GridUp-PCB (Autodesk Fusion 360 design; units mm, degrees)
part number: 2026-09-14-08-15-55-205
Autodesk Fusion 360 part; units mm, degrees
sketch "Çizim257" plane through (0, 0, 0) normal (0, 0, 1) x (1, 0, 0)
  line L0 (0, 0) -> (110, 0)
  line L1 (110, 0) -> (110, 70)
  line L2 (110, 70) -> (0, 70)
  line L3 (0, 70) -> (0, 0)
extrude "Ekstrüzyon257" add sketch "Çizim257" along normal blind 1.6 makes body 1
fillet "Kavis8" radius 2 4 edges at (0, 70, 0.8) (110, 70, 0.8) (110, 0, 0.8) (0, 0, 0.8) on bodies 1
sketch "Çizim258" plane through (0, 0, 0) normal (0, 0, 1) x (1, 0, 0)
  circle A0 centre (7, 7) radius 1.6
  circle A1 centre (103, 7) radius 1.6
  circle A2 centre (7, 63) radius 1.6
  circle A3 centre (103, 63) radius 1.6
  line L0 (81.5, -1) -> (82.5, -1)
  line L1 (82.5, -1) -> (82.5, 40)
  line L2 (82.5, 40) -> (81.5, 40)
  line L3 (81.5, 40) -> (81.5, -1)
  circle A4 centre (0, 0) radius 4
  circle A5 centre (110, 0) radius 4
  circle A6 centre (0, 70) radius 4
  circle A7 centre (110, 70) radius 4
extrude "Ekstrüzyon258" cut sketch "Çizim258" along normal mid plane 10 bodies 1
ref_plane "WorkPlane238" through (0, 0, 1.6) normal (0, 0, 1) x (1, 0, 0)
sketch "Çizim259" plane through (0, 0, 1.6) normal (0, 0, 1) x (1, 0, 0)
  circle A0 centre (55, 37.5) radius 4.65
extrude "Ekstrüzyon259" add sketch "Çizim259" along normal blind 6 separate body makes body 2
ref_plane "WorkPlane239" through (0, 0, 1.6) normal (0, 0, 1) x (1, 0, 0)
sketch "Çizim260" plane through (0, 0, 1.6) normal (0, 0, 1) x (1, 0, 0)
  line L0 (5.75, 29.75) -> (8.25, 29.75)
  line L1 (8.25, 29.75) -> (8.25, 32.25)
  line L2 (8.25, 32.25) -> (5.75, 32.25)
  line L3 (5.75, 32.25) -> (5.75, 29.75)
extrude "Ekstrüzyon260" add sketch "Çizim260" along normal blind 0.9 separate body makes body 3
ref_plane "WorkPlane240" through (0, 0, 1.6) normal (0, 0, 1) x (1, 0, 0)
sketch "Çizim261" plane through (0, 0, 1.6) normal (0, 0, 1) x (1, 0, 0)
  circle A0 centre (25, 65) radius 1.5
extrude "Ekstrüzyon261" add sketch "Çizim261" along normal blind 1.5 separate body makes body 4
ref_plane "WorkPlane241" through (0, 0, 1.6) normal (0, 0, 1) x (1, 0, 0)
sketch "Çizim262" plane through (0, 0, 1.6) normal (0, 0, 1) x (1, 0, 0)
  line L0 (37.5, 45.5) -> (39.5, 45.5)
  line L1 (39.5, 45.5) -> (39.5, 46.5)
  line L2 (39.5, 46.5) -> (37.5, 46.5)
  line L3 (37.5, 46.5) -> (37.5, 45.5)
extrude "Ekstrüzyon262" add sketch "Çizim262" along normal blind 0.6 separate body makes body 5
ref_plane "WorkPlane242" through (0, 0, 1.6) normal (0, 0, 1) x (1, 0, 0)
sketch "Çizim263" plane through (0, 0, 1.6) normal (0, 0, 1) x (1, 0, 0)
  line L0 (37.5, 43.75) -> (39.5, 43.75)
  line L1 (39.5, 43.75) -> (39.5, 44.75)
  line L2 (39.5, 44.75) -> (37.5, 44.75)
  line L3 (37.5, 44.75) -> (37.5, 43.75)
extrude "Ekstrüzyon263" add sketch "Çizim263" along normal blind 0.6 separate body makes body 6
ref_plane "WorkPlane243" through (0, 0, 1.6) normal (0, 0, 1) x (1, 0, 0)
sketch "Çizim264" plane through (0, 0, 1.6) normal (0, 0, 1) x (1, 0, 0)
  line L0 (37.5, 42) -> (38.75, 42)
  line L1 (38.75, 42) -> (38.75, 43)
  line L2 (38.75, 43) -> (37.5, 43)
  line L3 (37.5, 43) -> (37.5, 42)
extrude "Ekstrüzyon264" add sketch "Çizim264" along normal blind 0.6 separate body makes body 7
ref_plane "WorkPlane244" through (0, 0, 1.6) normal (0, 0, 1) x (1, 0, 0)
sketch "Çizim265" plane through (0, 0, 1.6) normal (0, 0, 1) x (1, 0, 0)
  line L0 (29, 51.5) -> (31, 51.5)
  line L1 (31, 51.5) -> (31, 52.5)
  line L2 (31, 52.5) -> (29, 52.5)
  line L3 (29, 52.5) -> (29, 51.5)
extrude "Ekstrüzyon265" add sketch "Çizim265" along normal blind 0.6 separate body makes body 8
ref_plane "WorkPlane245" through (0, 0, 1.6) normal (0, 0, 1) x (1, 0, 0)
sketch "Çizim266" plane through (0, 0, 1.6) normal (0, 0, 1) x (1, 0, 0)
  line L0 (29, 50) -> (31, 50)
  line L1 (31, 50) -> (31, 51)
  line L2 (31, 51) -> (29, 51)
  line L3 (29, 51) -> (29, 50)
extrude "Ekstrüzyon266" add sketch "Çizim266" along normal blind 0.6 separate body makes body 9
ref_plane "WorkPlane246" through (0, 0, 1.6) normal (0, 0, 1) x (1, 0, 0)
sketch "Çizim267" plane through (0, 0, 1.6) normal (0, 0, 1) x (1, 0, 0)
  line L0 (32, 49.75) -> (35, 49.75)
  line L1 (35, 49.75) -> (35, 52.75)
  line L2 (35, 52.75) -> (32, 52.75)
  line L3 (32, 52.75) -> (32, 49.75)
extrude "Ekstrüzyon267" add sketch "Çizim267" along normal blind 2 separate body makes body 10
ref_plane "WorkPlane247" through (0, 0, 0) normal (0, 0, 1) x (1, 0, 0)
sketch "Çizim268" plane through (0, 0, 0) normal (0, 0, 1) x (1, 0, 0)
  line L0 (10, 40.8) -> (28, 40.8)
  line L1 (28, 40.8) -> (28, 60)
  line L2 (28, 60) -> (10, 60)
  line L3 (10, 60) -> (10, 40.8)
extrude "Ekstrüzyon268" add sketch "Çizim268" against normal blind 3.2 separate body makes body 11
ref_plane "WorkPlane248" through (0, 0, 0) normal (0, 0, 1) x (1, 0, 0)
sketch "Çizim269" plane through (0, 0, 0) normal (0, 0, 1) x (1, 0, 0)
  line L0 (64, 42) -> (95.7, 42)
  line L1 (95.7, 42) -> (95.7, 68.7)
  line L2 (95.7, 68.7) -> (64, 68.7)
  line L3 (64, 68.7) -> (64, 42)
extrude "Ekstrüzyon269" add sketch "Çizim269" against normal blind 21.8 separate body makes body 12
ref_plane "WorkPlane249" through (0, 0, 0) normal (0, 0, 1) x (1, 0, 0)
sketch "Çizim270" plane through (0, 0, 0) normal (0, 0, 1) x (1, 0, 0)
  line L0 (88, 22.25) -> (94.1, 22.25)
  line L1 (94.1, 22.25) -> (94.1, 25)
  line L2 (94.1, 25) -> (88, 25)
  line L3 (88, 25) -> (88, 22.25)
extrude "Ekstrüzyon270" add sketch "Çizim270" against normal blind 2.6 separate body makes body 13
ref_plane "WorkPlane250" through (0, 0, 0) normal (0, 0, 1) x (1, 0, 0)
sketch "Çizim271" plane through (0, 0, 0) normal (0, 0, 1) x (1, 0, 0)
  line L0 (96.5, 21.5) -> (103.5, 21.5)
  line L1 (103.5, 21.5) -> (103.5, 25.5)
  line L2 (103.5, 25.5) -> (96.5, 25.5)
  line L3 (96.5, 25.5) -> (96.5, 21.5)
extrude "Ekstrüzyon271" add sketch "Çizim271" against normal blind 8 separate body makes body 14
ref_plane "WorkPlane251" through (0, 0, 0) normal (0, 0, 1) x (1, 0, 0)
sketch "Çizim272" plane through (0, 0, 0) normal (0, 0, 1) x (1, 0, 0)
  line L0 (84, 0.5) -> (99.25, 0.5)
  line L1 (99.25, 0.5) -> (99.25, 8.5)
  line L2 (99.25, 8.5) -> (84, 8.5)
  line L3 (84, 8.5) -> (84, 0.5)
extrude "Ekstrüzyon272" add sketch "Çizim272" against normal blind 10 separate body makes body 15
ref_plane "WorkPlane252" through (0, 0, 0) normal (0, 0, 1) x (1, 0, 0)
sketch "Çizim273" plane through (0, 0, 0) normal (0, 0, 1) x (1, 0, 0)
  line L0 (70, 34) -> (76.5, 34)
  line L1 (76.5, 34) -> (76.5, 41)
  line L2 (76.5, 41) -> (70, 41)
  line L3 (70, 41) -> (70, 34)
extrude "Ekstrüzyon273" add sketch "Çizim273" against normal blind 1.7 separate body makes body 16
ref_plane "WorkPlane253" through (0, 0, 0) normal (0, 0, 1) x (1, 0, 0)
sketch "Çizim274" plane through (0, 0, 0) normal (0, 0, 1) x (1, 0, 0)
  line L0 (76.75, 39) -> (81, 39)
  line L1 (81, 39) -> (81, 41.65)
  line L2 (81, 41.65) -> (76.75, 41.65)
  line L3 (76.75, 41.65) -> (76.75, 39)
extrude "Ekstrüzyon274" add sketch "Çizim274" against normal blind 1.5 separate body makes body 17
ref_plane "WorkPlane254" through (0, 0, 0) normal (0, 0, 1) x (1, 0, 0)
sketch "Çizim275" plane through (0, 0, 0) normal (0, 0, 1) x (1, 0, 0)
  line L0 (76.75, 35) -> (81, 35)
  line L1 (81, 35) -> (81, 37.65)
  line L2 (81, 37.65) -> (76.75, 37.65)
  line L3 (76.75, 37.65) -> (76.75, 35)
extrude "Ekstrüzyon275" add sketch "Çizim275" against normal blind 1.5 separate body makes body 18
ref_plane "WorkPlane255" through (0, 0, 0) normal (0, 0, 1) x (1, 0, 0)
sketch "Çizim276" plane through (0, 0, 0) normal (0, 0, 1) x (1, 0, 0)
  line L0 (60.5, 44.5) -> (62.5, 44.5)
  line L1 (62.5, 44.5) -> (62.5, 45.5)
  line L2 (62.5, 45.5) -> (60.5, 45.5)
  line L3 (60.5, 45.5) -> (60.5, 44.5)
extrude "Ekstrüzyon276" add sketch "Çizim276" against normal blind 0.6 separate body makes body 19
ref_plane "WorkPlane256" through (0, 0, 0) normal (0, 0, 1) x (1, 0, 0)
sketch "Çizim277" plane through (0, 0, 0) normal (0, 0, 1) x (1, 0, 0)
  line L0 (77.5, 29.5) -> (79.5, 29.5)
  line L1 (79.5, 29.5) -> (79.5, 30.5)
  line L2 (79.5, 30.5) -> (77.5, 30.5)
  line L3 (77.5, 30.5) -> (77.5, 29.5)
extrude "Ekstrüzyon277" add sketch "Çizim277" against normal blind 0.6 separate body makes body 20
ref_plane "WorkPlane257" through (0, 0, 0) normal (0, 0, 1) x (1, 0, 0)
sketch "Çizim278" plane through (0, 0, 0) normal (0, 0, 1) x (1, 0, 0)
  line L0 (77.5, 28) -> (79.5, 28)
  line L1 (79.5, 28) -> (79.5, 29)
  line L2 (79.5, 29) -> (77.5, 29)
  line L3 (77.5, 29) -> (77.5, 28)
extrude "Ekstrüzyon278" add sketch "Çizim278" against normal blind 0.6 separate body makes body 21
ref_plane "WorkPlane258" through (0, 0, 0) normal (0, 0, 1) x (1, 0, 0)
sketch "Çizim279" plane through (0, 0, 0) normal (0, 0, 1) x (1, 0, 0)
  line L0 (43.5, 36) -> (46, 36)
  line L1 (46, 36) -> (46, 38)
  line L2 (46, 38) -> (43.5, 38)
  line L3 (43.5, 38) -> (43.5, 36)
extrude "Ekstrüzyon279" add sketch "Çizim279" against normal blind 1 separate body makes body 22
ref_plane "WorkPlane259" through (0, 0, 0) normal (0, 0, 1) x (1, 0, 0)
sketch "Çizim280" plane through (0, 0, 0) normal (0, 0, 1) x (1, 0, 0)
  line L0 (43.5, 31.5) -> (46.5, 31.5)
  line L1 (46.5, 31.5) -> (46.5, 34.5)
  line L2 (46.5, 34.5) -> (43.5, 34.5)
  line L3 (43.5, 34.5) -> (43.5, 31.5)
extrude "Ekstrüzyon280" add sketch "Çizim280" against normal blind 1.5 separate body makes body 23
ref_plane "WorkPlane260" through (0, 0, 0) normal (0, 0, 1) x (1, 0, 0)
sketch "Çizim281" plane through (0, 0, 0) normal (0, 0, 1) x (1, 0, 0)
  line L0 (48, 26) -> (50, 26)
  line L1 (50, 26) -> (50, 27)
  line L2 (50, 27) -> (48, 27)
  line L3 (48, 27) -> (48, 26)
extrude "Ekstrüzyon281" add sketch "Çizim281" against normal blind 0.6 separate body makes body 24
ref_plane "WorkPlane261" through (0, 0, 0) normal (0, 0, 1) x (1, 0, 0)
sketch "Çizim282" plane through (0, 0, 0) normal (0, 0, 1) x (1, 0, 0)
  line L0 (48, 28.5) -> (50, 28.5)
  line L1 (50, 28.5) -> (50, 29.5)
  line L2 (50, 29.5) -> (48, 29.5)
  line L3 (48, 29.5) -> (48, 28.5)
extrude "Ekstrüzyon282" add sketch "Çizim282" against normal blind 0.6 separate body makes body 25
ref_plane "WorkPlane262" through (0, 17.75, 0) normal (0, 1, 0) x (0, 0, 1)
sketch "Çizim283" plane through (0, 17.75, 0) normal (0, 1, 0) x (1, 0, 0)
  circle A0 centre (61, 5.25) radius 5.25
extrude "Ekstrüzyon283" add sketch "Çizim283" along normal mid plane 31.5 separate body makes body 26
sketch "Çizim284" plane through (0, 17.75, 0) normal (0, 1, 0) x (1, 0, 0)
  circle A0 centre (72, 5.25) radius 5.25
extrude "Ekstrüzyon284" add sketch "Çizim284" along normal mid plane 31.5 separate body makes body 27
ref_plane "WorkPlane263" through (0, 0, 0) normal (0, 0, 1) x (1, 0, 0)
sketch "Çizim285" plane through (0, 0, 0) normal (0, 0, 1) x (1, 0, 0)
  line L0 (41.25, 14) -> (46.25, 14)
  line L1 (46.25, 14) -> (46.25, 20)
  line L2 (46.25, 20) -> (41.25, 20)
  line L3 (41.25, 20) -> (41.25, 14)
extrude "Ekstrüzyon285" add sketch "Çizim285" against normal blind 1.5 separate body makes body 28
ref_plane "WorkPlane264" through (0, 0, 0) normal (0, 0, 1) x (1, 0, 0)
sketch "Çizim286" plane through (0, 0, 0) normal (0, 0, 1) x (1, 0, 0)
  line L0 (47.5, 15) -> (48.5, 15)
  line L1 (48.5, 15) -> (48.5, 17)
  line L2 (48.5, 17) -> (47.5, 17)
  line L3 (47.5, 17) -> (47.5, 15)
extrude "Ekstrüzyon286" add sketch "Çizim286" against normal blind 0.6 separate body makes body 29
ref_plane "WorkPlane265" through (0, 0, 0) normal (0, 0, 1) x (1, 0, 0)
sketch "Çizim287" plane through (0, 0, 0) normal (0, 0, 1) x (1, 0, 0)
  line L0 (1, 11) -> (9, 11)
  line L1 (9, 11) -> (9, 26.25)
  line L2 (9, 26.25) -> (1, 26.25)
  line L3 (1, 26.25) -> (1, 11)
extrude "Ekstrüzyon287" add sketch "Çizim287" against normal blind 10 separate body makes body 30
ref_plane "WorkPlane266" through (0, 0, 0) normal (0, 0, 1) x (1, 0, 0)
sketch "Çizim288" plane through (0, 0, 0) normal (0, 0, 1) x (1, 0, 0)
  line L0 (25, 14) -> (27, 14)
  line L1 (27, 14) -> (27, 15)
  line L2 (27, 15) -> (25, 15)
  line L3 (25, 15) -> (25, 14)
extrude "Ekstrüzyon288" add sketch "Çizim288" against normal blind 0.6 separate body makes body 31
ref_plane "WorkPlane267" through (0, 0, 0) normal (0, 0, 1) x (1, 0, 0)
sketch "Çizim289" plane through (0, 0, 0) normal (0, 0, 1) x (1, 0, 0)
  line L0 (28, 14) -> (30, 14)
  line L1 (30, 14) -> (30, 15)
  line L2 (30, 15) -> (28, 15)
  line L3 (28, 15) -> (28, 14)
extrude "Ekstrüzyon289" add sketch "Çizim289" against normal blind 0.6 separate body makes body 32
ref_plane "WorkPlane268" through (0, 0, 0) normal (0, 0, 1) x (1, 0, 0)
sketch "Çizim290" plane through (0, 0, 0) normal (0, 0, 1) x (1, 0, 0)
  line L0 (31, 14) -> (33, 14)
  line L1 (33, 14) -> (33, 15)
  line L2 (33, 15) -> (31, 15)
  line L3 (31, 15) -> (31, 14)
extrude "Ekstrüzyon290" add sketch "Çizim290" against normal blind 0.6 separate body makes body 33
ref_plane "WorkPlane269" through (0, 0, 0) normal (0, 0, 1) x (1, 0, 0)
sketch "Çizim291" plane through (0, 0, 0) normal (0, 0, 1) x (1, 0, 0)
  line L0 (34, 14) -> (36, 14)
  line L1 (36, 14) -> (36, 15)
  line L2 (36, 15) -> (34, 15)
  line L3 (34, 15) -> (34, 14)
extrude "Ekstrüzyon291" add sketch "Çizim291" against normal blind 0.6 separate body makes body 34
ref_plane "WorkPlane270" through (0, 0, 0) normal (0, 0, 1) x (1, 0, 0)
sketch "Çizim292" plane through (0, 0, 0) normal (0, 0, 1) x (1, 0, 0)
  line L0 (37, 13) -> (39, 13)
  line L1 (39, 13) -> (39, 15)
  line L2 (39, 15) -> (37, 15)
  line L3 (37, 15) -> (37, 13)
extrude "Ekstrüzyon292" add sketch "Çizim292" against normal blind 0.6 separate body makes body 35
ref_plane "WorkPlane271" through (0, 0, 0) normal (0, 0, 1) x (1, 0, 0)
sketch "Çizim293" plane through (0, 0, 0) normal (0, 0, 1) x (1, 0, 0)
  line L0 (25, 0.5) -> (53, 0.5)
  line L1 (53, 0.5) -> (53, 7.5)
  line L2 (53, 7.5) -> (25, 7.5)
  line L3 (25, 7.5) -> (25, 0.5)
extrude "Ekstrüzyon293" add sketch "Çizim293" against normal blind 9 separate body makes body 36
ref_plane "WorkPlane272" through (0, 0, 0) normal (0, 0, 1) x (1, 0, 0)
sketch "Çizim294" plane through (0, 0, 0) normal (0, 0, 1) x (1, 0, 0)
  line L0 (11, 6.25) -> (24, 6.25)
  line L1 (24, 6.25) -> (24, 11.25)
  line L2 (24, 11.25) -> (11, 11.25)
  line L3 (11, 11.25) -> (11, 6.25)
extrude "Ekstrüzyon294" add sketch "Çizim294" against normal blind 8.5 separate body makes body 37
equation "d1045 = -( 3.2 mm )"
equation "d1049 = -( 21.8 mm )"
equation "d1053 = -( 2.6 mm )"
equation "d1057 = -( 8 mm )"
equation "d1061 = -( 10 mm )"
equation "d1065 = -( 1.7 mm )"
equation "d1069 = -( 1.5 mm )"
equation "d1073 = -( 1.5 mm )"
equation "d1077 = -( 0.6 mm )"
equation "d1081 = -( 0.6 mm )"
equation "d1085 = -( 0.6 mm )"
equation "d1089 = -( 1 mm )"
equation "d1093 = -( 1.5 mm )"
equation "d1097 = -( 0.6 mm )"
equation "d1101 = -( 0.6 mm )"
equation "d1111 = -( 1.5 mm )"
equation "d1115 = -( 0.6 mm )"
equation "d1119 = -( 10 mm )"
equation "d1123 = -( 0.6 mm )"
equation "d1127 = -( 0.6 mm )"
equation "d1131 = -( 0.6 mm )"
equation "d1135 = -( 0.6 mm )"
equation "d1139 = -( 0.6 mm )"
equation "d1143 = -( 9 mm )"
equation "d1147 = -( 8.5 mm )"
named bodies: "PCB", "MLX90640", "SHT31", "LED", "R_pullup1", "R_pullup2", "C_100n", "EN_RC1", "EN_RC2", "Reset", "ESP32-S3-WROOM-1U", "RAC05-05SK", "F1", "MOV", "Klemens 230V", "LDO SOT-223", "D1", "D2", "R_sarj", "Bolucu1", "Bolucu2", "Boost U7", "L_boost", "R_bal1", "R_bal2", "Superkap1", "Superkap2", "MAX3485", "R120", "Klemens RS-485", "R_burden1", "R_burden2", "R_burden3", "R_burden4", "R_bias", "Klemens CT", "Genisleme 2x5"
